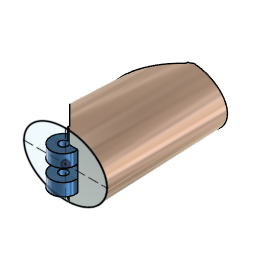
middle finger part 1 v3 (Autodesk Fusion 360 design; units mm, degrees)
Autodesk Fusion 360 part; units mm, degrees
sketch "base" plane through (0, 0, 0) normal (0, 1, 0) x (1, 0, 0)
  ellipse E0 centre (0, 0) end of major axis (10, 0) minor radius 7.5
  line L0 (-10, 0) -> (10, 0) construction
  line L1 (0, -7.5) -> (0, 7.5) construction
  dimension "d1" = 20
  dimension "d2" = 15
  constraint coincident E0 L0.start
  constraint coincident E0 L0.end
  constraint coincident E0 L1.start
  constraint coincident E0 L1.end
  constraint coincident E0.centre origin
  constraint horizontal L0
  measures "d1" distance of E0
ref_plane "WorkPlane1" through (0, 30, 0) normal (0, 1, 0) x (1, 0, 0)
sketch "top" plane through (0, 30, 0) normal (0, 1, 0) x (1, 0, 0)
  ellipse E0 centre (0, 0) end of major axis (9, 0) minor radius 6.5
  line L0 (-9, 0) -> (9, 0) construction
  line L1 (0, -6.5) -> (0, 6.5) construction
  dimension "d4" = 18
  dimension "d5" = 13
  constraint coincident E0 L0.start
  constraint coincident E0 L0.end
  constraint coincident E0 L1.start
  constraint coincident E0 L1.end
  constraint coincident E0.centre origin
  constraint horizontal L0
  measures "d4" distance of E0
loft "Loft1" add profiles "top", "base" section 1 section 2 makes body 1
sketch "cut" plane through (0, 0, 0) normal (0, 0, 1) x (1, 0, 0)
  line L0 (0, 30) -> (0, 30.5)
  line L1 (0, 0) -> (0, 1)
  line L2 (0, 1) -> (-14.1421, 15.1421)
  line L3 (0, 1) -> (20, 1) construction
  line L4 (-14.1421, 15.1421) -> (-14.1421, 0)
  line L5 (-14.1421, 0) -> (0, 0)
  line L6 (0, 0) -> (0, -0.5)
  line L7 (0, 30) -> (0, 29)
  line L8 (0, 29) -> (-14.1421, 14.8579)
  line L9 (0, 29) -> (20, 29) construction
  line L10 (0, 30) -> (-11.4565, 30)
  line L11 (-11.4565, 30) -> (-14.1421, 14.8579)
  dimension "d6" = 0.5
  dimension "d7" = 1
  dimension "d8" = 135
  dimension "d9" = 20
  dimension "d10" = 0.5
  dimension "d11" = 1
  dimension "d12" = 135
  dimension "d13" = 20
  constraint vertical L0
  constraint coincident L1.start L5.end
  constraint vertical L1
  constraint horizontal L3
  constraint parallel L1 L4
  constraint perpendicular L1 L5
  constraint perpendicular L5 L6
  constraint parallel L0 L7
  constraint horizontal L9
  constraint perpendicular L7 L10
  measures "d6" distance of L0.start L0.end
  measures "d7" distance of L1.start L1.end
  measures "d8" angle of L2 L3
  measures "d9" distance of L1.end L2.end
  measures "d10" distance of L1.start L6.end
  measures "d11" distance of L0.start L7.end
  measures "d12" angle of L8 L9
  measures "d13" distance of L7.end L8.end
extrude "Extrude1" cut sketch "cut" along normal mid plane 40 contours L1 L2 L4 L5 L8 | L2 L7 L8 L10 L11 bodies 1
sketch "wheel" plane through (0, 0, 0) normal (0, 0, 1) x (1, 0, 0)
  line L0 (0, 0) -> (0, -0.5)
  circle A0 centre (0, -0.5) radius 3
  circle A1 centre (0.0423, 30.5794) radius 3
  dimension "d16" = 0.5
  dimension "d17" = 6
  dimension "d18" = 6
  constraint coincident L0.start origin
  constraint vertical L0
  constraint coincident L0.end A0.centre
  measures "d16" distance of L0.start L0.end
  measures "d17" diameter of A0
  measures "d18" diameter of A1
extrude "Extrude2" add sketch "wheel" along normal mid plane 3 separate body contours A1 makes body 2
extrude "Extrude3" cut sketch "wheel" along normal mid plane 3 contours A0 bodies 1
sketch "lower wheel offset" plane through (0, 0, -1.5) normal (0, 0, 1) x (-1, 0, 0)
  line L0 (0, 0) -> (-2.958, 0)
  arc A0 (-2.958, 0) -> (1.2343, -2.2343) centre (0, 0.5) ccw
  line L1 (1.2343, -2.2343) -> (0, -1)
  line L2 (0, -1) -> (0, 0)
  circle A1 centre (0, 0.5) radius 3
  dimension "d23" = 6
  constraint concentric A0 A1
  measures "d23" diameter of A1
extrude "Extrude4" add sketch "lower wheel offset" against normal blind 3 separate body makes body 3
sketch "lower wheel offset2" plane through (0, 0, 1.5) normal (0, 0, -1) x (1, 0, 0)
  line L0 (2.958, 0) -> (0, 0)
  line L1 (0, 0) -> (0, -1)
  line L2 (0, -1) -> (-1.2343, -2.2343)
  arc A0 (-1.2343, -2.2343) -> (2.958, 0) centre (0, 0.5) ccw
  circle A1 centre (0, 0.5) radius 3
  dimension "d26" = 6
  constraint concentric A0 A1
  measures "d26" diameter of A1
extrude "Extrude5" add sketch "lower wheel offset2" against normal blind 3 separate body makes body 4
sketch "rod cut" plane through (0, 0, 0) normal (0, 0, 1) x (1, 0, 0)
  circle A0 centre (0, -0.5) radius 1
  circle A1 centre (0, 30.5) radius 1
  dimension "d29" = 2
  dimension "d30" = 2
  measures "d29" diameter of A0
  measures "d30" diameter of A1
extrude "Extrude6" cut sketch "rod cut" along normal mid plane 40 bodies 1 2 3 4
sketch "cut1" plane through (0, 0, 0) normal (0, 0, 1) x (1, 0, 0)
  line L0 (-9.1313, 28.0047) -> (-10.1313, 0.0047)
  line L1 (-9.3731, 21.234) -> (-9.8728, 21.2519)
  line L2 (-9.8728, 21.2519) -> (-10.3432, 8.0801)
  line L3 (-10.3432, 8.0801) -> (-7.8448, 7.9908)
  line L4 (-7.8448, 7.9908) -> (-7.3142, 22.8494)
  line L5 (-7.3142, 22.8494) -> (-9.5, 21.2405)
  dimension "d34" = 0.5
  dimension "d35" = 2.5
  constraint coincident L0 L1.start
  constraint perpendicular L0 L1
  constraint perpendicular L1 L2
  constraint perpendicular L0 L3
  constraint perpendicular L3 L4
  measures "d34" distance of L1.start L1.end
  measures "d35" distance of L2.end L3.end
extrude "Extrude7" cut sketch "cut1" along normal mid plane 2 contours L0 L3 L4 L5 | L0 L1 L2 L3 bodies 1
sketch "cut 2" plane through (0, 0, 0) normal (0, 0, 1) x (1, 0, 0)
  line L0 (-9, 28) -> (-10, 0)
  line L1 (-9.2187, 21.8761) -> (-8.719, 21.8582)
  line L2 (-8.719, 21.8582) -> (-9.1005, 11.1785)
  line L3 (-9.1005, 11.1785) -> (-8.1011, 11.1428)
  line L4 (-8.1011, 11.1428) -> (-7.7659, 20.5294)
  line L5 (-7.7659, 20.5294) -> (-8.719, 21.8582)
  dimension "d38" = 0.5
  dimension "d39" = 1
  constraint coincident L0 L1.start
  constraint perpendicular L0 L1
  constraint perpendicular L1 L2
  constraint perpendicular L2 L3
  constraint perpendicular L3 L4
  measures "d38" distance of L1.start L1.end
  measures "d39" distance of L2.end L3.end
extrude "Extrude8" cut sketch "cut 2" along normal mid plane 4 bodies 1
copy_body "Body->Comp1" bodies 1 removing the originals makes body 5 in component "index part 1"
copy_body "Body->Comp2" bodies 2 removing the originals makes body 6 in component "uppr wheel"
copy_body "Body->Comp3" bodies 3 removing the originals makes body 7 in component "lower wheel 1"
copy_body "Body->Comp4" bodies 4 removing the originals makes body 8 in component "lower wheel 2"
sketch "Sketch11" plane through (0, 0, 0) normal (0, 1, 0) x (1, 0, 0)
extrude "Extrude1'" cut 1 faces at (0.7378, 32.769, 1.5) along direction (0, 0, 1) blind 3 on bodies 6 bodies 5 in component "index part 1"
extrude "Extrude2'" cut 1 faces at (0.7378, 32.769, -1.5) along direction (0, 0, -1) blind 3 on bodies 6 bodies 5 in component "index part 1"
combine "Combine1" operation add target body 5 tool bodies 8 7 6 in component "index part 1"
component "index part 1" placed x (1, 0, 0) y (0, 1, 0) z (0, 0, 1) at (0, 0, 0)
component "uppr wheel" placed x (1, 0, 0) y (0, 1, 0) z (0, 0, 1) at (0, 0, 0)
component "lower wheel 1" placed x (1, 0, 0) y (0, 1, 0) z (0, 0, 1) at (0, 0, 0)
component "lower wheel 2" placed x (1, 0, 0) y (0, 1, 0) z (0, 0, 1) at (0, 0, 0)
named bodies: "index part 1", "uppr wheel", "lower wheel 1", "lower wheel 2"
